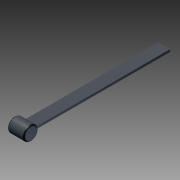
# Autodesk Inventor part: JointD2_2nd
Saved by Autodesk Inventor 2013 (Build 170138000, 138)
## iProperties
Created: 2013-02-07
Part Number: JointD2_2nd
Document SubType Name: Modeling
Designer: arihon
Density: 2.71 g/cm^3
Material: アルミニウム 6061
Mass: 1.30353 g
Surface Area: 8.69395 cm^2
Volume: 0.481008 cm^3
Author: arihon
Autodesk Inventor part; units mm, degrees
ref_plane "YZ Plane" through (0, 0, 0) normal (1, 0, 0) x (0, 1, 0)
ref_plane "XZ Plane" through (0, 0, 0) normal (0, 1, 0) x (-1, 0, 0)
ref_plane "XY Plane" through (0, 0, 0) normal (0, 0, 1) x (1, 0, 0)
sketch "スケッチ1" plane through (0, 0, 0) normal (0, 0, 1) x (1, 0, 0)
  line L0 (-2.5, 23.7333) -> (2.5, 23.7333)
  line L1 (2.5, 23.7333) -> (2.5, -36.2667)
  line L2 (2.5, -36.2667) -> (-2.5, -36.2667)
  line L3 (-2.5, -36.2667) -> (-2.5, 23.7333)
  point P0 (0, 0)
  dimension "d0" = 5
  dimension "d1" = 2.5
  dimension "d2" = 60
  constraints: 8 end point, 2 parallel, 1 horizontal, 1 perpendicular
  measures "d0" distance of L0.start L0.end
  measures "d1" distance from line of L3 point (0, 0)
  measures "d2" distance of L0.end L1.end
extrude "押し出し1" add sketch "スケッチ1" along normal blind 1
sketch "スケッチ2" plane through (0, 0, 1) normal (0, 0, 1) x (1, 0, 0)
  line L0 (2.5, 23.7333) -> (2.5, -36.2667) projected
  line L1 (-2.5, -36.2667) -> (2.5, -36.2667)
  line L2 (2.5, -36.2667) -> (2.5, -33.2667)
  line L3 (2.5, -33.2667) -> (-2.5, -33.2667)
  line L4 (-2.5, -33.2667) -> (-2.5, -36.2667)
  point P0 (0, 0)
  dimension "d5" = 3
  constraints: 8 end point, 2 parallel, 1 horizontal, 1 perpendicular, 1 point on line
  measures "d5" distance between parallel lines of L1 L3
extrude "押し出し2" cut sketch "スケッチ2" against normal blind 0.5
sketch "スケッチ4" plane through (0, 0, 0.5) normal (0, 0, 1) x (1, 0, 0)
  line L0 (2.5, -33.2667) -> (2.5, -36.2667) projected
  line L1 (2.5, -36.2667) -> (-2.5, -36.2667) projected
  line L2 (-3.5, -33.2667) -> (3.5, -33.2667)
  line L3 (3.5, -33.2667) -> (3.5, -36.2667)
  line L4 (3.5, -36.2667) -> (-3.5, -36.2667)
  line L5 (-3.5, -36.2667) -> (-3.5, -33.2667)
  point P0 (0, 0)
  dimension "d9" = 7
  dimension "d10" = 1
  constraints: 8 end point, 2 parallel, 1 horizontal, 1 perpendicular, 1 point on line
  measures "d9" distance between parallel lines of L5 L3
  measures "d10" distance between parallel lines of L3 L0
revolve "回転2" add sketch "スケッチ4" angle 360 about axis through (2.5, -36.2667, 0.5) along (-1, 0, 0)
fillet "フィレット1" radius 0.5 2 edges at (-3.5, -39.2667, 0.5) (3.5, -39.2667, 0.5)
equation "\"d1\" = 0.5 * d0"
